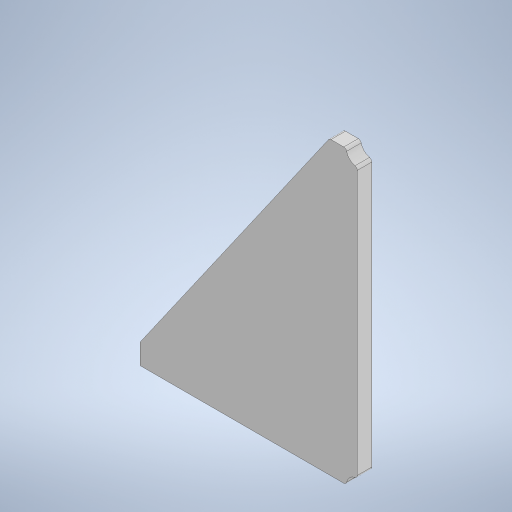
# Autodesk Inventor part: Costilla (rib)
Saved by Autodesk Inventor 2024.3 (Build 283343000, 343)
## iProperties
Created: 2025-07-04
Part Number: Costilla (rib)
Material: Genérico
Document SubType Name: Modeling
Designer: Daniel Rodriguez
Density: 1 g/cm^3
Appearance: Valor por defecto
Author: Daniel Rodriguez
Autodesk Inventor part; units mm, degrees
ref_plane "YZ Plane" through (0, 0, 0) normal (1, 0, 0) x (0, 1, 0)
ref_plane "XZ Plane" through (0, 0, 0) normal (0, 1, 0) x (-1, 0, 0)
ref_plane "XY Plane" through (0, 0, 0) normal (0, 0, 1) x (1, 0, 0)
sketch "Boceto1" plane through (0, 0, 0) normal (0, 0, 1) x (1, 0, 0)
  line L0 (0, 0) -> (149.172, 0)
  line L1 (149.172, 0) -> (149.172, 200)
  line L2 (0, 14) -> (0, 0)
  line L3 (149.172, 200) -> (130, 200)
  line L4 (130, 200) -> (0, 14)
  arc A0 (149.172, 7.5) -> (141.672, 0) centre (149.172, 0) ccw
  arc A1 (141.672, 200) -> (149.172, 192.5) centre (149.172, 200) ccw
  line L5 (0, 0) -> (141.672, 0) construction
  line L6 (-4.7533, 0) -> (0, 0) construction
  dimension "d1" = 149.172
  dimension "d2" = 200
  dimension "d3" = 7.5
  dimension "d4" = 7.5
  dimension "d13" = 14
  dimension "d14" = 130
  constraints: 14 end point, 4 point on circle, 4 point on line, 3 horizontal, 2 centre point, 2 coincident, 2 perpendicular, 1 vertical
  measures "d1" distance of L0.start L0.end
  measures "d2" distance of L0.end L1.end
  measures "d3" radius of A0
  measures "d4" radius of A1
  measures "d13" distance of L2.start L0.start
  measures "d14" horizontal distance of L3.end L2.start
extrude "Extrusión1" add sketch "Boceto1" along normal mid plane 10 contours L2 L4 L3 A1 L1 A0 L0
fillet "Empalme1" radius 2 6 edges at (149.172, 7.5, 0) (141.672, 0, 0) (149.172, 192.5, 0) (141.672, 200, 0) (130, 200, 0) (0, 14, 0)
